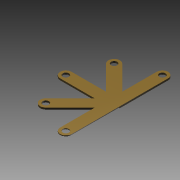
# Autodesk Inventor part: HS13Z-trmnls
Saved by Autodesk Inventor 2011 SP1 (Build 150282100, 282)
## iProperties
Created: 2016-09-01
Part Number: HS13Z-trmnls
Catalog Web Link: www.cadenas.de
Description: HS Series - 6 AMP Single Pole Standard Size Rotaries -trmnls-
Vendor: NKKSWITCHES
Document SubType Name: Modeling
Designer: psAdmin
Manufacturer: NKKSWITCHES
Mass: 0.284842 g
Surface Area: 10.5169 cm^2
Volume: 0.284842 cm^3
Density: 1 g/cm^3
Category: PARTsolutions
Company: NKKSWITCHES
Title: HS13Z-trmnls
Author: Cadenas PARTsolutions
PSOL_IDENT_0: {$CADENAS_DATA\23d-libs\nkkswitches\rotary\hs_12_amp\parts\hs_6amp_terminals.prj},220 {VTYP=3D},{NB=
PSOL_IDENT_1: HS13Z-trmnls},{LINA=HS13Z-trmnls},{NN=HS Series - 6 AMP Single Pole Standard Size Rotaries -trmnls},
PSOL_IDENT_2: {DATE=22.09.2015 06:04:15},{GEOMDATE=02.04.2009 06:58:00},{VERSION=},{LINEID=30},{LINESUBID=-1},{WBV
PSOL_IDENT_3: AR=}  {NB=HS13Z-trmnls},{LINA=HS13Z-trmnls},{KT=DUMMY},{PN=HS13Z},{SRS=HS},{MDL=HS13Z},{NP=4}
NN: HS Series - 6 AMP Single Pole Standard Size Rotaries -trmnls
NB: HS13Z-trmnls
NBSYN: $PN.-trmnls
LINA: HS13Z-trmnls
PN: HS13Z
SRS: HS
MDL: HS13Z
NP: 4
SUPPLIER: NKKSWITCHES
ARTICLENO: HS13Z-trmnls
BOMINFO: HS13Z-trmnls
CREATOR: CADENAS GmbH
Autodesk Inventor part; units mm, degrees
sketch "Sketch_1" plane through (0, 0, 0) normal (0, 1, 0) x (-1, 0, 0)
  arc A0 (2.4003, 20.2946) -> (-2.4003, 20.2946) centre (0, 20.2946) ccw
  line L0 (-2.4003, 20.2946) -> (-2.4003, 0)
  line L1 (-2.4003, 0) -> (2.4003, 0)
  line L2 (2.4003, 0) -> (2.4003, 20.2946)
  circle A1 centre (0, 20.2946) radius 1.2954
  constraints: 6 end point, 2 centre point, 2 point on circle
extrude "Extrusion1" add sketch "Sketch_1" against normal blind 0.3048
sketch "Sketch_2" plane through (0, 0, 0) normal (0, 1, 0) x (-1, 0, 0)
  arc A0 (16.0477, 12.6532) -> (12.6532, 16.0477) centre (14.3504, 14.3504) ccw
  line L0 (12.6532, 16.0477) -> (-1.6973, 1.6973)
  line L1 (-1.6973, 1.6973) -> (1.6973, -1.6973)
  line L2 (1.6973, -1.6973) -> (16.0477, 12.6532)
  circle A1 centre (14.3504, 14.3504) radius 1.2954
  constraints: 6 end point, 2 centre point, 2 point on circle
extrude "Extrusion2" add sketch "Sketch_2" against normal blind 0.7112
sketch "Sketch_3" plane through (0, 0, 0) normal (0, 1, 0) x (-1, 0, 0)
  arc A0 (20.2946, -2.4003) -> (20.2946, 2.4003) centre (20.2946, 0) ccw
  line L0 (20.2946, 2.4003) -> (0, 2.4003)
  line L1 (0, 2.4003) -> (0, -2.4003)
  line L2 (0, -2.4003) -> (20.2946, -2.4003)
  circle A1 centre (20.2946, 0) radius 1.2954
  constraints: 6 end point, 2 centre point, 2 point on circle
extrude "Extrusion3" add sketch "Sketch_3" against normal blind 0.7112
sketch "Sketch_4" plane through (0, 0, 0) normal (0, 1, 0) x (-1, 0, 0)
  arc A0 (12.6532, -16.0477) -> (16.0477, -12.6532) centre (14.3504, -14.3504) ccw
  line L0 (16.0477, -12.6532) -> (1.6973, 1.6973)
  line L1 (1.6973, 1.6973) -> (-1.6973, -1.6973)
  line L2 (-1.6973, -1.6973) -> (12.6532, -16.0477)
  circle A1 centre (14.3504, -14.3504) radius 1.2954
  constraints: 6 end point, 2 centre point, 2 point on circle
extrude "Extrusion4" add sketch "Sketch_4" against normal blind 0.7112
sketch "Sketch_5" plane through (0, 0, 0) normal (0, 1, 0) x (-1, 0, 0)
  line L0 (2.4003, -20.2946) -> (2.4003, 0)
  line L1 (2.4003, 0) -> (-2.4003, 0)
  line L2 (-2.4003, 0) -> (-2.4003, -20.2946)
  arc A0 (-2.4003, -20.2946) -> (2.4003, -20.2946) centre (0, -20.2946) ccw
  circle A1 centre (0, -20.2946) radius 1.2954
  constraints: 6 end point, 2 centre point, 2 point on circle
extrude "Extrusion5" add sketch "Sketch_5" against normal blind 0.7112
ref_plane "to_body_XY" through (0, 0, 0) normal (0, -1, 0) x (1, 0, 0)
ref_plane "to_body_YZ" through (0, 0, 0) normal (1, 0, 0) x (0, 0, 1)
ref_plane "to_body_ZX" through (0, 0, 0) normal (0, 0, 1) x (0, -1, 0)
body "Solid1"
